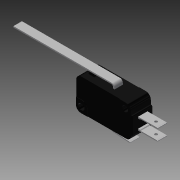
# Autodesk Inventor part: V7-2B17D8-048
Saved by Autodesk Inventor 2014 (Build 180170000, 170)
## iProperties
Category: Sensors
Company: Autodesk, Inc.
Created: 2013-12-21
Part Number: V7-2B17D8-048
Document SubType Name: Modeling
Project: FIRST
Catalog Web Link: http://sensing.honeywell.com/index.php?ci_id=3108&la_id=1&pr_id=29368
Description: Switch - Snap Action Basic
Vendor: Honeywell
Surface Area: 27.6054 cm^2
Volume: 4.47812 cm^3
Material: Generic
Designer: Autodesk, Inc.
Appearance: Glossy - Black
Title: Switch - Snap Action Basic
Author: Autodesk, Inc.
Autodesk Inventor part; units mm, degrees
ref_plane "YZ Plane" through (0, 0, 0) normal (1, 0, 0) x (0, 1, 0)
ref_plane "XZ Plane" through (0, 0, 0) normal (0, 1, 0) x (-1, 0, 0)
ref_plane "XY Plane" through (0, 0, 0) normal (0, 0, 1) x (1, 0, 0)
sketch "Sketch1" plane through (0, 0, 0) normal (0, 0, 1) x (1, 0, 0)
  line L0 (93.6182, 164.6593) -> (88.4158, 164.6593)
  line L1 (126.1074, 112.8426) -> (126.1074, 118.0049)
  line L2 (101.092, 59.4863) -> (101.092, 74.0504)
  line L3 (101.092, 56.175) -> (101.092, 51.9605)
  line L4 (101.092, 48.9501) -> (101.092, 43.8325)
  line L5 (77.2674, 164.6593) -> (58.5793, 164.6593)
  line L6 (77.2674, 154.4485) -> (58.514, 154.4485)
  line L7 (140.1921, 173.0458) -> (140.1921, 182.7972)
  line L8 (99.8761, 164.6593) -> (80.4039, 164.6593)
  line L9 (99.0589, 76.3067) -> (108.7131, 76.3067)
  line L10 (99.8293, 154.4485) -> (93.3707, 154.4485)
  line L11 (100.0068, 154.4485) -> (80.5999, 154.4485)
  line L12 (126.1074, 87.3057) -> (126.1074, 91.3759)
  line L13 (130.4036, 182.7972) -> (130.4036, 174.9485)
  line L14 (126.1074, 87.0115) -> (126.1074, 86.3739)
  line L15 (99.8388, 76.3067) -> (75.8918, 76.3067)
  line L16 (125.844, 69.4161) -> (125.844, 66.4266)
  line L17 (65.2158, 97.5779) -> (55.8407, 97.5779)
  line L18 (130.4036, 171.1978) -> (130.4036, 162.5594)
  line L19 (119.5197, 147.6322) -> (116.9797, 147.6322)
  line L20 (116.9797, 147.6322) -> (108.6725, 157.4924)
  line L21 (110.8, 154.9671) -> (108.6725, 157.4924)
  line L22 (102.2858, 74.6563) -> (102.2858, 55.8845)
  line L23 (105.4862, 74.7933) -> (105.4862, 56.0215)
  line L24 (103.886, 77.3282) -> (103.886, 80.0686)
  line L25 (162.9321, 89.3985) -> (166.9961, 89.3985)
  line L26 (139.8234, 76.336) -> (139.8234, 59.4445)
  line L27 (139.8234, 57.1797) -> (139.8234, 54.9149)
  line L28 (117.9032, 91.6242) -> (117.9032, 93.9927)
  line L29 (140.3529, 83.6587) -> (143.7236, 83.6587)
  line L30 (155.9278, 70.0205) -> (160.6983, 70.0205)
  line L31 (150.6268, 78.0707) -> (156.7155, 78.0707)
  line L32 (121.85, 86.6051) -> (130.3648, 86.6051)
  line L33 (126.1074, 85.9571) -> (126.1074, 83.1619)
  line L34 (103.886, 75.3414) -> (103.886, 69.381)
  line L35 (150.7016, 77.5627) -> (163.4748, 77.5627)
  line L36 (140.4366, 78.0707) -> (148.6464, 78.0707)
  line L37 (140.5309, 77.5627) -> (148.7408, 77.5627)
  line L38 (127.8163, 89.3985) -> (148.4545, 89.3985)
  line L39 (155.9055, 83.6587) -> (163.5339, 83.6587)
  line L40 (139.8234, 82.6933) -> (139.8234, 78.8765)
  line L41 (146.503, 83.6587) -> (154.3088, 83.6587)
  line L42 (129.921, 48.9501) -> (129.921, 43.8325)
  line L43 (126.1074, 105.0993) -> (126.1074, 110.2615)
  line L44 (139.3042, 70.0205) -> (130.7168, 70.0205)
  line L45 (126.6197, 70.0205) -> (129.329, 70.0205)
  line L46 (140.4366, 70.0205) -> (154.3084, 70.0205)
  line L47 (129.921, 84.9342) -> (129.921, 86.0635)
  line L48 (129.921, 56.175) -> (129.921, 51.9605)
  line L49 (151.2487, 89.3985) -> (160.6983, 89.3985)
  line L50 (162.9321, 73.4981) -> (166.9961, 73.4981)
  line L51 (127.5604, 73.4981) -> (129.0656, 73.4981)
  line L52 (139.2098, 73.4981) -> (130.5281, 73.4981)
  line L53 (140.4366, 73.4981) -> (154.3084, 73.4981)
  line L54 (156.1175, 73.4981) -> (161.0645, 73.4981)
  line L55 (160.4589, 86.6051) -> (129.1173, 86.6051)
  line L56 (179.7148, 86.6051) -> (175.9519, 86.6051)
  line L57 (162.9321, 86.6051) -> (173.092, 86.6051)
  line L58 (134.8489, 104.3012) -> (132.3089, 104.3012)
  line L59 (132.3089, 104.3012) -> (118.7973, 104.2927)
  line L60 (118.7973, 104.2927) -> (125.0888, 87.7573)
  line L61 (123.9145, 90.8435) -> (125.0888, 87.7573)
  line L62 (126.1074, 74.9969) -> (126.1074, 63.9631)
  line L63 (129.921, 59.4863) -> (129.921, 76.5369)
  line L64 (126.1074, 90.2578) -> (126.1074, 103.4054)
  line L65 (129.921, 90.2578) -> (129.921, 103.4054)
  line L66 (129.921, 87.1121) -> (129.921, 88.8059)
  line L67 (128.905, 105.0993) -> (128.905, 110.2615)
  line L68 (128.905, 90.2578) -> (128.905, 103.4054)
  line L69 (128.905, 88.8059) -> (128.905, 88.08)
  line L70 (129.921, 105.0993) -> (129.921, 110.2615)
  circle A0 centre (126.1074, 86.6051) radius 1.4986
  line L71 (123.0594, 86.6051) -> (123.0594, 89.3985)
  line L72 (126.1074, 83.5571) -> (128.905, 83.5571)
  line L73 (129.921, 157.5981) -> (118.0302, 157.5981)
  line L74 (106.9304, 154.6517) -> (106.7272, 154.4485)
  line L75 (104.5675, 74.8589) -> (103.2044, 74.8589)
  arc A1 (103.2044, 77.7545) -> (103.2044, 74.8589) centre (103.886, 76.3067) ccw
  arc A2 (106.9375, 76.2915) -> (103.8895, 79.3395) centre (103.8895, 76.2915) ccw
  line L76 (66.4921, 157.3949) -> (66.4921, 161.7129)
  line L77 (106.9375, 76.2915) -> (106.9375, 73.4981)
  line L78 (103.8895, 79.3395) -> (101.0919, 79.3395)
  arc A3 (104.5675, 74.8589) -> (104.5675, 77.7545) centre (103.886, 76.3067) ccw
  line L79 (101.092, 164.6593) -> (101.092, 161.7129)
  line L80 (118.0302, 161.9923) -> (118.0302, 157.1155)
  line L81 (116.8872, 161.9923) -> (118.0302, 161.9923)
  line L82 (116.8872, 157.1155) -> (118.0302, 157.1155)
  line L83 (117.1784, 157.3949) -> (117.1784, 157.1155)
  line L84 (112.1882, 157.3949) -> (112.1882, 157.1155)
  line L85 (66.4921, 161.7129) -> (118.0302, 161.7129)
  line L86 (66.4921, 157.3949) -> (118.0302, 157.3949)
  line L87 (116.8872, 157.3949) -> (116.8872, 157.1155)
  line L88 (129.921, 83.6587) -> (139.0749, 83.6587)
  line L89 (126.365, 89.3985) -> (103.632, 89.3985)
  line L90 (139.0749, 77.5627) -> (129.921, 77.5627)
  line L91 (131.214, 78.0707) -> (139.0749, 78.0707)
  line L92 (103.6318, 73.4981) -> (126.365, 73.4981)
  line L93 (116.8872, 161.9923) -> (116.8872, 161.7129)
  line L94 (111.0452, 157.3949) -> (111.0452, 157.1155)
  line L95 (123.0594, 154.6517) -> (101.092, 154.6517)
  line L96 (128.905, 154.4485) -> (123.0594, 154.4485)
  line L97 (123.0594, 154.6517) -> (123.0594, 154.4485)
  line L98 (128.905, 154.6517) -> (129.921, 154.6517)
  line L99 (111.0452, 157.1155) -> (112.1882, 157.1155)
  line L100 (101.092, 157.3949) -> (101.092, 154.4485)
  line L101 (139.4436, 157.2933) -> (139.4436, 162.0431)
  line L102 (139.4436, 162.0431) -> (140.1921, 161.2831)
  line L103 (139.4436, 157.2933) -> (140.1921, 158.0534)
  line L104 (130.4036, 162.0431) -> (139.4436, 162.0431)
  line L105 (130.4036, 157.2933) -> (139.4436, 157.2933)
  circle A4 centre (137.0171, 159.6682) radius 0.6985
  line L106 (130.4036, 162.0431) -> (130.4036, 161.624)
  line L107 (130.4036, 161.624) -> (129.921, 161.624)
  line L108 (129.921, 157.7124) -> (130.4036, 157.7124)
  line L109 (130.4036, 157.7124) -> (130.4036, 157.2933)
  line L110 (106.7272, 154.4485) -> (101.092, 154.4485)
  line L111 (101.092, 164.6593) -> (106.9376, 164.6593)
  line L112 (140.1921, 158.0534) -> (140.1921, 161.2831)
  line L113 (66.4921, 91.6089) -> (116.4521, 91.6089)
  arc A5 (116.0791, 71.7289) -> (117.2561, 70.5579) centre (117.3455, 71.8248) ccw
  line L114 (66.4921, 90.9739) -> (116.3494, 90.9739)
  arc A6 (116.8872, 71.799) -> (117.5961, 71.0387) centre (117.6492, 71.7988) ccw
  line L115 (125.9079, 70.3174) -> (125.892, 70.0893)
  line L116 (119.5477, 70.3929) -> (119.5831, 70.8997)
  line L117 (116.0791, 71.7289) -> (115.8712, 71.7412)
  line L118 (66.4921, 91.6089) -> (66.4921, 90.9739)
  line L119 (116.9855, 90.3312) -> (117.1031, 89.3985)
  line L120 (117.6155, 90.4107) -> (117.7431, 89.3985)
  arc A7 (116.9855, 90.3312) -> (116.2403, 90.9978) centre (116.0984, 90.0893) ccw
  arc A8 (117.6155, 90.4107) -> (116.2493, 91.6328) centre (116.1816, 90.1824) ccw
  arc A9 (101.0919, 76.0381) -> (103.632, 73.4981) centre (103.6319, 76.0381) ccw
  arc A10 (103.632, 89.3985) -> (101.0919, 86.8585) centre (103.6319, 86.8585) ccw
  arc A11 (128.905, 86.8585) -> (126.365, 89.3985) centre (126.365, 86.8585) ccw
  arc A12 (126.365, 73.4981) -> (128.8946, 75.8081) centre (126.365, 76.0381) ccw
  arc A13 (129.921, 84.1902) -> (129.159, 84.9522) centre (129.159, 84.1902) ccw
  arc A14 (129.159, 76.2921) -> (129.921, 77.0541) centre (129.159, 77.0541) ccw
  line L121 (128.8946, 75.8081) -> (128.8946, 76.2921)
  line L122 (129.921, 77.0541) -> (129.921, 84.1902)
  line L123 (128.905, 86.8585) -> (128.905, 83.5571)
  line L124 (129.159, 76.2921) -> (128.8946, 76.2921)
  line L125 (128.905, 84.9522) -> (129.159, 84.9522)
  line L126 (129.921, 164.4561) -> (129.921, 154.6517)
  line L127 (101.0919, 86.8585) -> (101.0919, 76.0381)
  line L128 (104.5675, 77.7545) -> (103.2044, 77.7545)
  line L129 (128.905, 164.6593) -> (128.905, 154.4485)
  arc A15 (104.954, 90.7988) -> (104.4666, 90.0708) centre (105.4704, 89.9259) ccw
  arc A16 (106.7732, 90.7988) -> (104.954, 90.7988) centre (105.8636, 88.5913) ccw
  arc A17 (107.2606, 90.0708) -> (106.7732, 90.7988) centre (106.2568, 89.9259) ccw
  line L130 (104.4666, 90.0708) -> (104.4666, 89.3985)
  line L131 (107.2606, 90.0708) -> (107.2606, 89.3985)
  line L132 (123.0594, 164.6593) -> (128.905, 164.6593)
  line L133 (123.0594, 164.4561) -> (101.092, 164.4561)
  line L134 (117.1784, 161.9923) -> (117.1784, 161.7129)
  line L135 (123.0594, 164.4561) -> (123.0594, 164.6593)
  line L136 (129.921, 164.4561) -> (128.905, 164.4561)
  line L137 (111.0452, 161.9923) -> (111.0452, 161.7129)
  line L138 (139.8234, 83.5267) -> (139.8234, 83.2827)
  line L139 (139.0749, 83.6587) -> (139.8234, 83.5267)
  line L140 (139.0749, 83.1507) -> (139.8234, 83.2827)
  line L141 (111.0452, 161.9923) -> (112.1882, 161.9923)
  line L142 (131.214, 83.1507) -> (139.0749, 83.1507)
  line L143 (130.4036, 83.6587) -> (130.4036, 82.8459)
  line L144 (130.9092, 82.8459) -> (129.921, 82.8459)
  line L145 (112.1882, 161.7129) -> (112.1882, 161.9923)
  line L146 (139.0749, 83.1507) -> (139.0749, 83.6587)
  line L147 (130.9092, 82.8459) -> (131.214, 83.1507)
  line L148 (130.4036, 77.5627) -> (130.4036, 78.3755)
  line L149 (129.921, 78.3755) -> (130.9092, 78.3755)
  line L150 (130.9092, 78.3755) -> (131.214, 78.0707)
  line L151 (106.9376, 164.4561) -> (106.9376, 164.6593)
  line L152 (139.0749, 78.0707) -> (139.8234, 77.9387)
  line L153 (139.0749, 78.0707) -> (139.0749, 77.5627)
  line L154 (139.0749, 77.5627) -> (139.8234, 77.6947)
  line L155 (139.8234, 77.6947) -> (139.8234, 77.9387)
  line L156 (115.8712, 73.4981) -> (115.8712, 71.7412)
  line L157 (116.8872, 73.4981) -> (116.8872, 71.7986)
  line L158 (116.8872, 73.3744) -> (115.8712, 73.3744)
  arc A18 (123.0594, 86.6051) -> (126.1074, 83.5571) centre (126.1074, 86.6051) ccw
  line L159 (105.3706, 78.8457) -> (105.5281, 78.6882)
  line L160 (105.2808, 78.8457) -> (105.5473, 78.5792)
  line L161 (105.2045, 78.8323) -> (105.5253, 78.5114)
  line L162 (105.1525, 78.7945) -> (105.4983, 78.4486)
  line L163 (105.1004, 78.7567) -> (105.4463, 78.4108)
  line L164 (105.0758, 78.6915) -> (105.3943, 78.373)
  line L165 (105.0538, 78.6237) -> (105.315, 78.3626)
  line L166 (105.0782, 78.5095) -> (105.2252, 78.3626)
  line L167 (95.9775, 78.8096) -> (96.065, 78.7221)
  line L168 (95.8516, 78.8457) -> (96.1008, 78.5965)
  line L169 (95.7656, 78.8419) -> (96.0788, 78.5287)
  line L170 (95.7136, 78.8041) -> (96.0568, 78.4609)
  line L171 (95.6615, 78.7663) -> (96.0074, 78.4204)
  line L172 (95.6293, 78.7088) -> (95.9554, 78.3826)
  line L173 (95.6073, 78.641) -> (95.8857, 78.3626)
  line L174 (95.615, 78.5434) -> (95.7959, 78.3626)
  line L175 (125.9079, 70.3174) -> (125.144, 70.5109)
  line L176 (125.892, 70.0893) -> (125.1351, 70.007)
  line L177 (125.144, 70.5109) -> (117.5961, 71.0387)
  line L178 (125.1351, 70.007) -> (117.2561, 70.5579)
  point P0 (0, 0)
  point P1 (157.7113, 49.3175)
  point P2 (120.2454, 146.3622)
  point P3 (120.2454, 142.6127)
  point P4 (135.5746, 103.0312)
  dimension "d1" = 22.2214
  dimension "d3" = 28.829
  dimension "d5" = 10.2984
  dimension "d7" = 0
  dimension "d9" = 9.7885
  dimension "d11" = 15.3022
  dimension "d13" = 10.2108
  dimension "d15" = 6.096
  dimension "d17" = 16.5846
  dimension "d19" = 59.6153
  dimension "d21" = 0.508
  dimension "d23" = 3.175
  dimension "d25" = 4.7498
  dimension "d27" = 3.2004
  dimension "d29" = 5.969
  dimension "d31" = 0.2635
  dimension "d33" = 13.716
  dimension "d35" = 8.2042
  dimension "d37" = 2.8956
  dimension "d39" = 2.7934
  dimension "d41" = 2.9464
  dimension "d43" = 15.9004
  dimension "d45" = 1.016
  constraints: 358 end point, 63 point on line, 39 point on circle, 19 centre point, 4 midpoint, 1 parallel, 1 tangent, 4 other
  measures "d1" distance between parallel lines of L34 L62
  measures "d3" distance of L4.start L42.start
  measures "d5" vertical distance of L9.start L32.start
  measures "d7" distance from line of L80 L85.end
  measures "d9" distance from line of L13 L7.start
  measures "d11" vertical distance of L9.start L113.start
  measures "d13" distance between parallel lines of L10 L8
  measures "d15" vertical distance of L35.start L39.start
  measures "d17" vertical distance of L30.start L56.end
  measures "d19" horizontal distance of L113.start L1.start
  measures "d21" distance between parallel lines of L35 L31
  measures "d23" horizontal distance of A4.centre L102.end
  measures "d25" distance of L101.start L101.end
  measures "d27" distance between parallel lines of L22 L23
  measures "d29" vertical distance of L113.start L17.start
  measures "d31" distance from line of L16 L62.start
  measures "d33" horizontal distance of L62.start L27.start
  measures "d35" horizontal distance of L28.start L43.start
  measures "d37" distance of L75.end L128.end
  measures "d39" vertical distance of L32.end L89.start
  measures "d41" distance from line of L29 L32.end
  measures "d43" distance of L50.start L25.start
  measures "d45" distance of L67.start L70.start
extrude "Extrusion1" add sketch "Sketch1" along normal mid plane 9.8044 contours L127 L78 L24 L128 A1 L9 | L9 A1 L75 L34 L92 A9 L127 | A1 L128 A3 L9 | L9 A3 L75 A1 | L127 A10 L89 L71 A18 L72 L123 L125 A13 L122 A14 L124 L121 A12 L92 L77 A2 L78 | A3 L128 L24 L78 A2 L9 | L9 A2 L77 L92 L34 L75 A3 | L89 L12 A0 L32 L71 | L32 A0 L33 A18 | A0 L32 | L32 A0 | L33 A0 L32 L123 L72 | L89 A11 L123 L32 A0 L12
sketch "Sketch2" plane through (0, 0, 4.9022) normal (0, 0, 1) x (1, 0, 0)
  line L0 (103.632, 89.3985) -> (126.365, 89.3985) projected
  arc A0 (103.632, 89.3985) -> (101.0919, 86.8585) centre (103.6319, 86.8585) ccw projected
  line L1 (101.0919, 76.0381) -> (101.0919, 86.8585) projected
  arc A1 (101.0919, 76.0381) -> (103.6318, 73.4981) centre (103.6319, 76.0381) ccw projected
  line L2 (126.365, 73.4981) -> (103.6318, 73.4981) projected
  arc A2 (126.365, 73.4981) -> (128.8946, 75.8081) centre (126.365, 76.0381) ccw projected
  line L3 (128.8946, 76.2921) -> (128.8946, 75.8081) projected
  line L4 (129.159, 76.2921) -> (128.8946, 76.2921) projected
  arc A3 (129.159, 76.2921) -> (129.921, 77.0541) centre (129.159, 77.0541) ccw projected
  line L5 (129.921, 84.1902) -> (129.921, 77.0541) projected
  arc A4 (129.921, 84.1902) -> (129.159, 84.9522) centre (129.159, 84.1902) ccw projected
  line L6 (128.905, 84.9522) -> (129.159, 84.9522) projected
  line L7 (128.905, 86.8585) -> (128.905, 84.9522) projected
  arc A5 (128.905, 86.8585) -> (126.365, 89.3985) centre (126.365, 86.8585) ccw projected
  point P0 (0, 0)
extrude "Extrusion2" add sketch "Sketch1" along normal mid plane 10.2108 contours L127 L78 L24 L128 A1 L9 | L9 A1 L75 L34 L92 A9 L127 | A1 L128 A3 L9 | L9 A3 L75 A1 | A3 L128 L24 L78 A2 L9 | L9 A2 L77 L92 L34 L75 A3 | L89 L12 A0 L32 L71 | L32 A0 L33 A18 | A0 L32 | L32 A0 | L33 A0 L32 L123 L72 | L89 A11 L123 L32 A0 L12
extrude "Extrusion3" cut sketch "Sketch1" along normal through all both and the other way through all contours A1 L128 A3 L9 | L9 A3 L75 A1 | A0 L32 | L32 A0
extrude "Extrusion4" add sketch "Sketch1" along normal mid plane 3.81 contours L130 A15 A16 L114 A17 L131 L89 | A16 L114
extrude "Extrusion5" add sketch "Sketch1" along normal mid plane 4.318 contours L119 A7 L114 A16 L118 L113 A8 L120 L89 | A16 L114
extrude "Extrusion6" add sketch "Sketch1" along normal mid plane 4.7498 contours L92 L157 L158 L156 | L158 L157 A6 L177 L116 L178 A5 L117 L156 | L177 L175 L115 L176 L178 L116 | L122 L149 L148 L90 | L148 L149 L150 L91 L153 L90 | L88 L143 L144 L122 | L153 L152 L155 L154 | L88 L146 L142 L147 L144 L143 | L139 L138 L140 L146
hole "Hole1" at (136.6484, 83.6587, 0) direction (0, -1, 0) diameter 1.397 end through all
hole "Hole2" at (122.7153, 70.1762, 0) direction (0.0697565, 0.997564, 0) diameter 1.397 end up to surface
equation "\"d48\" = d13"
equation "\"d50\" = d13"
equation "\"d56\" = d25"
equation "\"d59\" = 0.5 * d25"
equation "\"d67\" = 0.5 * d25"
equation "\"d68\" = d23"
body "Solid1"
